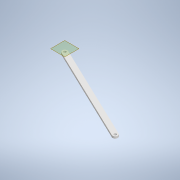
# Autodesk Inventor part: truss frame slanting
Saved by Autodesk Inventor 2020 (Build 240168000, 168)
## iProperties
Created: 2020-07-04
Part Number: truss frame slanting
Material: Generic
Document SubType Name: Modeling
Designer: Ashiqrahman
Density: 1 g/cm^3
Appearance: Default
Author: Ashiqrahman
Autodesk Inventor part; units mm, degrees
ref_plane "YZ Plane" through (0, 0, 0) normal (1, 0, 0) x (0, 1, 0)
ref_plane "XZ Plane" through (0, 0, 0) normal (0, 1, 0) x (-1, 0, 0)
ref_plane "XY Plane" through (0, 0, 0) normal (0, 0, 1) x (1, 0, 0)
ref_plane "Work Plane1" through (67.8546, -14.3758, -29.4077) normal (0, -1, 0) x (1, 0, 0)
sketch "Sketch1" plane through (67.8546, -14.3758, -29.4077) normal (0, -1, 0) x (1, 0, 0)
  line L0 (21.35, -30) -> (6.35, -30) projected
  arc A0 (26.35, -35) -> (21.35, -30) centre (21.35, -35) ccw projected
  line L1 (26.35, -50) -> (26.35, -35) projected
  circle A1 centre (20.4921, -35.8579) radius 2 projected
  line L2 (156.5537, 50) -> (166.162, 33.3579) projected
  arc A2 (166.162, 33.3579) -> (174.8223, 33.3579) centre (170.4921, 35.8579) ccw projected
  line L3 (174.8223, 33.3579) -> (184.4306, 50) projected
  circle A3 centre (170.4921, 35.8579) radius 2 projected
  line L4 (20.4921, -35.8579) -> (170.4921, 35.8579) construction
  line L5 (22.2175, -39.4666) -> (172.2175, 32.2491)
  line L6 (168.7668, 39.4666) -> (18.7668, -32.2491)
  arc A4 (18.7668, -32.2491) -> (22.2175, -39.4666) centre (20.4921, -35.8579) ccw
  arc A5 (172.2175, 32.2491) -> (168.7668, 39.4666) centre (170.4921, 35.8579) ccw
  point P0 (-67.8546, 29.4077)
  point P1 (95.4921, 0)
  dimension "d0" = 8
  constraints: 8 end point, 4 point on circle, 4 tangent, 2 centre point, 1 midpoint, 1 parallel
  measures "d0" diameter of A5
extrude "Extrusion1" add sketch "Sketch1" along normal blind 3
body "Solid1"
